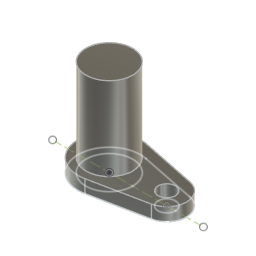
Hall Sensor v1 (Autodesk Fusion 360 design; units mm, degrees)
Autodesk Fusion 360 part; units mm, degrees
sketch "Sketch1" plane through (0, 0, 0) normal (0, 0, 1) x (1, 0, 0)
  circle A0 centre (22, 0) radius 3.3
  line L0 (2.38, 11.6596) -> (23.5, 7.3485)
  line L1 (36, 0) -> (-21.665, 0) construction
  line L2 (2.38, -11.6596) -> (23.5, -7.3485)
  arc A1 (23.5, -7.3485) -> (23.5, 7.3485) centre (22, 0) ccw
  arc A2 (2.38, 11.6596) -> (2.38, -11.6596) centre (0, 0) ccw
  circle A3 centre (0, 0) radius 8.93
  dimension "d1" = 23.8
  dimension "d2" = 15
  dimension "d3" = 22
  dimension "d4" = 6.6
  dimension "d5" = 17.86
  constraint coincident A2.centre A3.centre
  constraint concentric A0 A1
  constraint tangent L0 A2
  constraint horizontal L1
  constraint coincident A0.centre L1
  constraint tangent L0 A1
  constraint tangent L2 A2
  constraint tangent L2 A1
  measures "d1" diameter of A2
  measures "d2" diameter of A1
  measures "d3" distance of A2.centre A0.centre
  measures "d4" diameter of A0
  measures "d5" diameter of A3
extrude "Extrude1" add sketch "Sketch1" along normal blind 5
extrude "Extrude2" add sketch "Sketch1" along normal blind 36.75 contours A3
equation "d8 = 5 mm + 31.75 mm"
